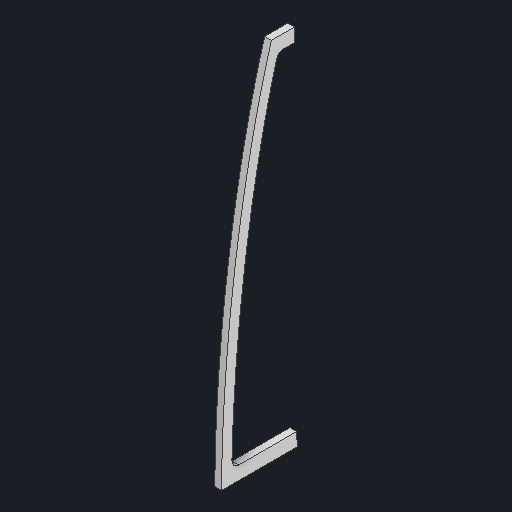
# Autodesk Inventor part: nose_spanner
Saved by Autodesk Inventor 2023 (Build 270158030, 158C)
## iProperties
Created: 2022-07-02
Part Number: nose_spanner
Material: Generic
Document SubType Name: Modeling
Designer: kardo
Density: 1 g/cm^3
Appearance: Default
Author: kardo
Autodesk Inventor part; units mm, degrees
ref_plane "YZ Plane" through (0, 0, 0) normal (1, 0, 0) x (0, 1, 0)
ref_plane "XZ Plane" through (0, 0, 0) normal (0, 1, 0) x (-1, 0, 0)
ref_plane "XY Plane" through (0, 0, 0) normal (0, 0, 1) x (1, 0, 0)
derived "surface_body.ipt"
sketch "sk_rail_top_tunnel" plane through (81.12, 0, 0) normal (1, 0, 0) x (0, 1, 0)
  line L0 (255, 107.6209) -> (255, -224.5198)
  line L1 (0, 107.6209) -> (0, -224.5198)
  line L2 (-345, 107.6209) -> (-345, -224.5198)
  line L3 (-345, 0) -> (0, 0)
  line L4 (-172.5, 48.8998) -> (-172.5, 0)
  line L5 (0, 52.89) -> (37.026, 52.89)
  line L6 (37.026, 52.89) -> (80.784, 47.0555)
  line L7 (80.784, 47.0555) -> (112.2, 37.536)
  line L8 (112.2, 107.6209) -> (112.2, -224.5198)
  line L9 (0, 52.89) -> (255, 52.89)
  line L10 (-469.9272, 0) -> (379.2584, 0)
  spline S0 degree 3 poles (0, 52.89) (92.8353, 52.89) (195.0311, 49.5089) (255, 36.448) knots 0 0 0 0 1 1 1 1
  spline S1 degree 3 poles (0, 52.89) (37.026, 52.89) (80.784, 47.0555) (112.2, 37.536) knots 1 1 1 1 2 2 2 2
  spline S2 degree 4 poles (-345, 37.4554) (-258.8682, 45.1562) (-172.5926, 49.7838) (-86.3161, 52.89) (0, 52.89) knots 0 0 0 0 0 1 1 1 1 1
  point P0 (153, 48.7795)
  point P1 (112.2, 28.832)
  point P2 (-230.0001, 45.8702)
  point P3 (-114.9999, 51.0173)
sketch "sk_rail_bottom_tunnel" plane through (81.12, 0, 0) normal (1, 0, 0) x (0, 1, 0)
  line L0 (-241.5001, 19.2432) -> (11.22, 28.376)
  arc A0 (36.465, 28.832) -> (11.22, 28.376) centre (36.465, -670.197) ccw
  line L1 (36.465, 28.832) -> (112.2, 28.832)
  arc A1 (-262.2001, 18.586) -> (-241.5001, 19.2432) centre (-326.8578, 2381.2399) ccw
  line L2 (-345, 16.32) -> (-262.2001, 18.586)
  point P0 (0, 0)
ref_plane "plane_tunnel_right" through (81.12, 0, 0) normal (1, 0, 0) x (0, 1, 0)
ref_plane "plane_middle" through (0, 0, 0) normal (0, 1, 0) x (-1, 0, 0)
derived "parameters_frame.ipt"
sketch "sk_base" plane through (81.12, 0, 0) normal (1, 0, 0) x (0, 1, 0)
  spline S0 degree 3 poles (0, 52.89) (37.026, 52.89) (80.784, 47.0555) (112.2, 37.536) knots 1 1 1 1 2 2 2 2 construction
  line L0 (36.465, 28.832) -> (112.2, 28.832) construction
  arc A0 (36.465, 28.832) -> (11.22, 28.376) centre (36.465, -670.197) ccw construction
  line L1 (-241.5001, 19.2432) -> (11.22, 28.376) construction
  line L2 (0, 3001.5237) -> (0, -1340.4629) construction
  line L3 (110.2, 36.8814) -> (110.2, 30.032)
  line L4 (110.2, 30.032) -> (106.2, 30.032)
  line L5 (106.2, 34.9098) -> (106.2, 30.032)
  line L6 (110.2, 30.032) -> (110.2, 28.832) construction
  line L7 (112.2, 37.536) -> (112.2, 28.832) construction
  line L8 (2, 51.6843) -> (2, 29.2436)
  line L9 (2, 29.2436) -> (6, 29.3881)
  line L10 (6, 29.3881) -> (6, 48.6396)
  line L11 (6, 29.3881) -> (6.0433, 28.1889)
  line L12 (2, 29.2436) -> (2.0433, 28.0444)
  spline S1 degree 5 poles (2, 51.6843) (13.2458, 51.621) (24.4883, 51.1202) (35.7087, 50.2782) (57.5045, 47.9978) (79.125, 44.4157) (89.5849, 42.338) (99.9758, 39.8957) (110.2, 36.8812) knots 0 0 0 0 0 0 0.513393 0.513393 0.513393 1 1 1 1 1 1
  spline S2 degree 5 poles (6, 48.6396) (16.3633, 48.4677) (26.7205, 47.938) (37.0577, 47.1181) (57.2276, 44.9624) (77.2464, 41.6841) (86.9805, 39.7913) (96.6556, 37.5847) (106.2, 34.9096) knots 0 0 0 0 0 0 0.511159 0.511159 0.511159 1 1 1 1 1 1
  point P0 (0, 0)
  dimension "d3" = 4.2
  dimension "d11" = 1.2
  dimension "d5" = 4
  dimension "d6" = 1.2
  dimension "d7" = 2
  dimension "d8" = 2
  dimension "d9" = 4
  dimension "d10" = 1.2
  constraints: 20 end point, 6 parallel, 3 perpendicular, 3 point on line, 6 other
  measures "d5" distance between parallel lines of L3 L5
  measures "d6" distance of L3.end L6.end
  measures "d7" distance between parallel lines of L7 L3
  measures "d8" distance between parallel lines of L2 L8
  measures "d9" distance between parallel lines of L8 L10
  measures "d10" distance of L9.end L11.end
extrude "Extrusion1" add sketch "sk_base" against normal blind 2
fillet "Fillet1" radius 2 2 edges at (80.12, 106.2, 34.9096) (80.12, 6, 48.6396)
equation "\"d3\" = shell_thickness + 0.75 * bulkhead_inset"
equation "\"d11\" = shell_thickness"
equation "\"d5\" = bulkhead_inset"
equation "\"d6\" = shell_thickness"
equation "\"d7\" = bulkhead_thickness"
equation "\"d8\" = bulkhead_thickness"
equation "\"d9\" = bulkhead_inset"
equation "\"d10\" = shell_thickness"
equation "\"d12\" = bulkhead_thickness"
equation "\"d14\" = 0.5 * bulkhead_inset"
equation "\"shell_thickness\" = 1.2"
equation "\"bulkhead_inset\" = 4"
equation "\"bulkhead_thickness\" = 2"
body "Solid1"
